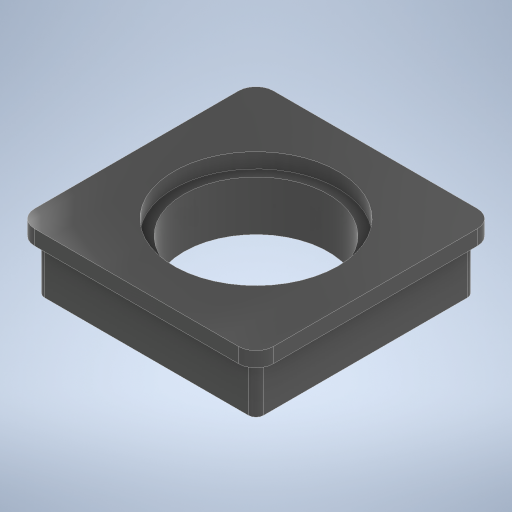
# Autodesk Inventor part: Cap_top
Saved by Autodesk Inventor 2023 (Build 270158000, 158)
## iProperties
Created: 2022-09-21
Part Number: Cap_top
Material: Стекло, литое, серое
Document SubType Name: Modeling
Designer: Makar
Density: 2.3 g/cm^3
Appearance: Темно-серый
Mass: 37.6977 g
Surface Area: 74.3996 cm^2
Volume: 16.3903 cm^3
Масса: 0.0
Author: Makar
Autodesk Inventor part; units mm, degrees
ref_plane "YZ Plane" through (0, 0, 0) normal (1, 0, 0) x (0, 1, 0)
ref_plane "XZ Plane" through (0, 0, 0) normal (0, 1, 0) x (-1, 0, 0)
ref_plane "XY Plane" through (0, 0, 0) normal (0, 0, 1) x (1, 0, 0)
sketch "Эскиз1" plane through (0, 0, 0) normal (0, 1, 0) x (-1, 0, 0)
  arc A0 (41, -50) -> (45.5, -45.5) centre (41, -45.5) ccw
  line L0 (0, -50) -> (41, -50)
  arc A1 (-4.5, -45.5) -> (0, -50) centre (0, -45.5) ccw
  line L1 (-4.5, -4.5) -> (-4.5, -45.5)
  arc A2 (0, 0) -> (-4.5, -4.5) centre (0, -4.5) ccw
  line L2 (-1.5, -45.5) -> (-1.5, -4.5)
  arc A3 (0, -3) -> (-1.5, -4.5) centre (0, -4.5) ccw
  line L3 (0, -3) -> (41, -3)
  line L4 (41, 0) -> (0, 0)
  arc A4 (45.5, -4.5) -> (41, 0) centre (41, -4.5) ccw
  line L5 (45.5, -45.5) -> (45.5, -4.5)
  line L6 (42.5, -4.5) -> (42.5, -45.5)
  arc A5 (42.5, -4.5) -> (41, -3) centre (41, -4.5) ccw
  line L7 (41, -47) -> (0, -47)
  arc A6 (41, -47) -> (42.5, -45.5) centre (41, -45.5) ccw
  arc A7 (-1.5, -45.5) -> (0, -47) centre (0, -45.5) ccw
  circle A8 centre (20.5, -25) radius 18.5
  circle A9 centre (20.5, -25) radius 16.5
  circle A10 centre (20.5, -25) radius 14.5
  circle A11 centre (20.5, -25) radius 13.5
  point P0 (11.5, -30)
  constraints: 16 end point, 16 point on circle, 12 centre point
extrude "Выдавливание1" add sketch "Эскиз1" along normal blind 10 contours L2 A3 L3 A5 L6 A6 L7 A7 | A8 | A9 | A10 | A11
extrude "Выдавливание2" cut sketch "Эскиз1" along normal blind 3 contours A8 | A10
extrude "Выдавливание3" cut sketch "Эскиз1" along normal blind 14.75 contours A10 | A11
extrude "Выдавливание4" add sketch "Эскиз1" along normal blind 13 contours L0 A1 L1 A2 L4 A4 L5 A0
extrude "Выдавливание5" add sketch "Эскиз1" along normal blind 13 contours L2 A3 L3 A5 L6 A6 L7 A7 | A8 | A9 | A10 | A11
extrude "Выдавливание6" cut sketch "Эскиз1" along normal blind 10 contours L0 A1 L1 A2 L4 A4 L5 A0
extrude "Выдавливание7" cut sketch "Эскиз1" along normal blind 3 contours A8 | A10
extrude "Выдавливание8" cut sketch "Эскиз1" along normal blind 15 contours A10 | A11
sketch "Эскиз2" plane through (0, 13, 0) normal (0, 1, 0) x (1, 0, 0)
  circle A0 centre (-20.5, 25) radius 14.5 projected
  line L0 (-45.5, 45.5) -> (-45.5, 4.5) projected
  arc A1 (-45.5, 4.5) -> (-41, 0) centre (-41, 4.5) ccw projected
  line L1 (-41, 0) -> (0, 0) projected
  arc A2 (0, 0) -> (4.5, 4.5) centre (0, 4.5) ccw projected
  line L2 (4.5, 4.5) -> (4.5, 45.5) projected
  arc A3 (4.5, 45.5) -> (0, 50) centre (0, 45.5) ccw projected
  line L3 (0, 50) -> (-41, 50) projected
  arc A4 (-41, 50) -> (-45.5, 45.5) centre (-41, 45.5) ccw projected
  circle A5 centre (-20.5, 25) radius 16.5
  constraints: 1 centre point, 1 coincident
extrude "Выдавливание9" cut sketch "Эскиз2" against normal blind 3 contours A5
sketch "Эскиз3" plane through (0, 13, 0) normal (0, 1, 0) x (1, 0, 0)
  circle A0 centre (-20.5, 25) radius 16.5 projected
  line L0 (-45.5, 45.5) -> (-45.5, 4.5) projected
  arc A1 (-45.5, 4.5) -> (-41, 0) centre (-41, 4.5) ccw projected
  line L1 (-41, 0) -> (0, 0) projected
  arc A2 (0, 0) -> (4.5, 4.5) centre (0, 4.5) ccw projected
  line L2 (4.5, 4.5) -> (4.5, 45.5) projected
  arc A3 (4.5, 45.5) -> (0, 50) centre (0, 45.5) ccw projected
  line L3 (0, 50) -> (-41, 50) projected
  arc A4 (-41, 50) -> (-45.5, 45.5) centre (-41, 45.5) ccw projected
  line L4 (-41, 49) -> (0, 49)
  arc A5 (3.5, 45.5) -> (0, 49) centre (0, 45.5) ccw
  line L5 (3.5, 45.5) -> (3.5, 4.5)
  arc A6 (0, 1) -> (3.5, 4.5) centre (0, 4.5) ccw
  line L6 (0, 1) -> (-41, 1)
  arc A7 (-44.5, 4.5) -> (-41, 1) centre (-41, 4.5) ccw
  line L7 (-44.5, 4.5) -> (-44.5, 45.5)
  arc A8 (-41, 49) -> (-44.5, 45.5) centre (-41, 45.5) ccw
  dimension "d18" = 1
  constraints: 8 end point, 8 point on circle, 4 centre point, 7 other
  measures "d18" distance between parallel lines of L3 L4
extrude "Выдавливание10" cut sketch "Эскиз3" against normal blind 3 contours A4 L3 A3 L2 A2 L1 A1 L0
